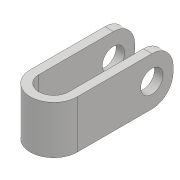
# Autodesk Inventor part: Suspension_Clamp_U-Clevis
Saved by Autodesk Inventor 2018 (Build 220112000, 112)
## iProperties
Created: 2021-04-28
Part Number: Suspension_Clamp_U-Clevis
Material: Generic
Document SubType Name: Modeling
Designer: l01767
Density: 1 g/cm^3
Appearance: Default
Author: l01767
Autodesk Inventor part; units mm, degrees
ref_plane "YZ Plane" through (0, 0, 0) normal (1, 0, 0) x (0, 1, 0)
ref_plane "XZ Plane" through (0, 0, 0) normal (0, 1, 0) x (-1, 0, 0)
ref_plane "XY Plane" through (0, 0, 0) normal (0, 0, 1) x (1, 0, 0)
sketch "Sketch1" plane through (0, 0, 0) normal (0, 0, 1) x (1, 0, 0)
  arc A0 (-14, 0) -> (14, 0) centre (0, 0) ccw
  line L0 (-14, 0) -> (-14, 90)
  line L1 (-14, 90) -> (-22, 90)
  line L2 (-22, 90) -> (-22, 0)
  arc A1 (-22, 0) -> (22, 0) centre (0, 0) ccw
  line L3 (0, 0) -> (0, -14)
  line L4 (14, 0) -> (14, 90)
  line L5 (14, 90) -> (22, 90)
  line L6 (22, 90) -> (22, 0)
  dimension "d0" = 14
  dimension "d1" = 90
  dimension "d2" = 8
  constraints: 14 end point, 5 point on circle, 2 centre point, 2 coincident, 2 horizontal alignment, 2 symmetric about line, 2 tangent, 1 horizontal, 1 perpendicular, 1 vertical
  measures "d0" radius of A0
  measures "d1" distance of L0.start L0.end
  measures "d2" distance between parallel lines of L0 L2
extrude "Extrusion1" add sketch "Sketch1" along normal mid plane 45
hole "Hole1" at (22, 70, 0) direction (-1, 0, 0) diameter 21 end through all
fillet "Fillet1" radius 20 4 edges at (18, 90, 22.5) (18, 90, -22.5) (-18, 90, -22.5) (-18, 90, 22.5)
body "Solid1"
